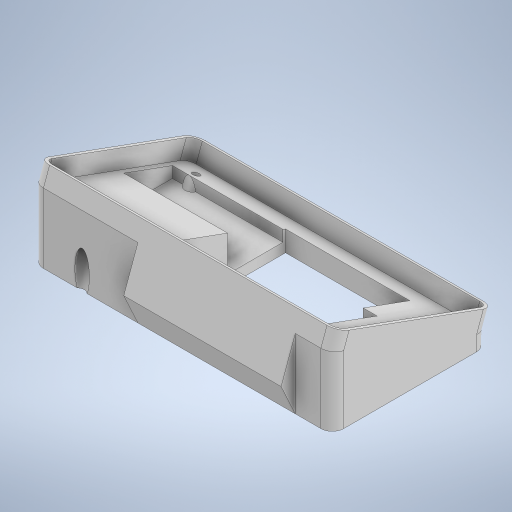
# Autodesk Inventor part: 5inDisplayAdapter-OLED-v3
Saved by Autodesk Inventor 2023 (Build 270158000, 158)
## iProperties
Created: 2024-03-13
Part Number: 5inDisplayAdapter-OLED-v3
Material: Generic
Document SubType Name: Modeling
Designer: incep
Density: 1 g/cm^3
Appearance: Default
Author: incep
## iProperties of the stored document 5inDisplayAdapter_3DPrint.ipt
Created: 2024-03-13
Part Number: 5inDisplayAdapter_3DPrint
Material: Generic
Document SubType Name: Modeling
Designer: incep
Density: 1 g/cm^3
Appearance: Default
Author: incep
Autodesk Inventor part; units mm, degrees
ref_plane "YZ Plane" through (0, 0, 0) normal (1, 0, 0) x (0, 1, 0)
sketch "Sketch1" plane through (0, 0, 0) normal (0, 1, 0) x (-1, 0, 0)
  circle A0 centre (32.29, -13) radius 2.1
  circle A1 centre (-62.1, -13) radius 2.1
  line L0 (72.5, -43) -> (-72.5, -43)
  line L1 (-72.5, -43) -> (-72.5, 32)
  line L2 (-72.5, 32) -> (72.5, 32)
  line L3 (72.5, 32) -> (72.5, -43)
  line L4 (15.095, -33) -> (-44.905, -33)
  line L5 (-44.905, -33) -> (-44.905, 7)
  line L6 (-44.905, 7) -> (15.095, 7)
  line L7 (15.095, 7) -> (15.095, -33)
  line L8 (-62.1, -13) -> (32.29, -13) construction
  point P0 (0, 0)
  point P1 (0, 0)
  point P2 (-14.905, -33)
  point P3 (0, -43)
  point P4 (-44.905, -13)
  point P5 (-72.5, -5.5)
  point P6 (15.095, -13)
  point P7 (-14.905, 7)
  point P8 (0, 32)
  point P9 (-14.905, -13)
  dimension "d1" = 4.2
  dimension "d2" = 60
  dimension "d3" = 40
  dimension "d55" = 25
  dimension "d56" = 10
  dimension "d76" = 145
  dimension "d77" = 75
  dimension "d78" = 94.39
  dimension "d107" = 10.4
  constraints: 18 end point, 8 midpoint, 4 parallel, 3 coincident, 3 horizontal, 2 centre point, 2 perpendicular, 2 vertical alignment, 1 horizontal alignment
  measures "d1" diameter of A0
  measures "d2" distance of L4.start L4.end
  measures "d3" distance between parallel lines of L4 L6
  measures "d55" distance between parallel lines of L2 L6
  measures "d56" distance between parallel lines of L0 L4
  measures "d76" distance of L1.end L2.end
  measures "d77" distance of L0.end L1.end
  measures "d78" distance of L8.start L8.end
  measures "d107" distance from line of L1 A1.centre
extrude "Extrusion1" add sketch "Sketch1" along normal blind 1
sketch "Sketch6" plane through (0, 0, 0) normal (1, 0, 0) x (0, 1, 0)
  line L0 (0, 32) -> (33.618656, 32)
  line L1 (33.618656, 32) -> (6.257045, -43.17541)
  line L2 (0, -43) -> (1, -43)
  line L3 (6.257045, -43.17541) -> (0, -43)
  line L4 (0, -43) -> (0, 32)
  line L5 (0, 32) -> (1, 32)
  line L6 (28.297768, 32) -> (0.9899, -43.027751)
  point P0 (0, 0)
  dimension "d15" = 70
  dimension "d16" = 80
  dimension "d25" = 5
  constraints: 10 end point, 3 point on line, 1 collinear, 1 parallel, 1 perpendicular
  measures "d15" angle of L1 L0
  measures "d16" distance of L0.end L1.end
  measures "d25" distance between parallel lines of L1 L6
extrude "Extrusion2" add sketch "Sketch6" along normal up to surface (72.5 mm away)
sketch "Sketch7" plane through (72.5, 0, 32) normal (1, 0, 0) x (0, 0, -1)
  line L0 (0, 0) -> (75, 0)
  line L1 (75.17541, 6.257045) -> (75, 0)
  line L2 (0, 33.618656) -> (75.17541, 6.257045)
  line L3 (0, 0) -> (0, 33.618656)
  point P0 (32, 0)
extrude "Extrusion3" add sketch "Sketch7" against normal up to surface (145 mm away)
sketch "Sketch8" plane through (-56.5, 6.257045, -43.17541) normal (0, 0.9396926, -0.3420201) x (1, 0, 0)
  line L0 (101.405, -45.009427) -> (41.405, -45.009427) construction
  line L1 (101.405, -7.421722) -> (101.405, -45.009427) construction
  line L2 (41.405, -7.421722) -> (101.405, -7.421722) construction
  line L3 (41.405, -45.009427) -> (41.405, -7.421722) construction
  ellipse E0 centre (24.21, -26.215574) end of major axis (22.11, -26.215574) minor radius 1.973355 construction
  ellipse E1 centre (118.6, -26.215574) end of major axis (116.5, -26.215574) minor radius 1.973355 construction
  line L4 (-3.875, -8.625) -> (118.125, -8.625) construction
  line L5 (118.125, -8.625) -> (118.125, -56.325) construction
  line L6 (118.125, -56.325) -> (-3.875, -56.325) construction
  line L7 (-3.875, -56.325) -> (-3.875, -8.625) construction
  line L8 (-16, 0) -> (129, 0) construction
  circle A0 centre (-3.875, -8.625) radius 1.75
  circle A1 centre (118.125, -8.625) radius 1.75
  circle A2 centre (118.125, -56.325) radius 1.75
  circle A3 centre (-3.875, -56.325) radius 1.75 construction
  line L9 (-16, -80) -> (129, -80)
  line L10 (129, -80) -> (129, 0)
  line L11 (-16, 0) -> (-16, -80)
  line L12 (-3.875, -8.625) -> (8.175, -8.625) construction
  line L13 (8.175, -8.625) -> (8.175, -71.075) construction
  line L14 (8.175, -71.075) -> (-3.875, -71.075) construction
  line L15 (-3.875, -71.075) -> (-3.875, -8.625) construction
  circle A4 centre (8.175, -71.075) radius 1.75
  line L16 (127.5, -1.5) -> (-14.5, -1.5)
  line L17 (-14.5, -1.5) -> (-14.5, -78.5)
  line L18 (-14.5, -78.5) -> (127.5, -78.5)
  line L19 (127.5, -78.5) -> (127.5, -1.5)
  circle A5 centre (8.175, -71.075) radius 3.5
  circle A6 centre (-3.875, -8.625) radius 3.5
  circle A7 centre (118.125, -8.625) radius 3.5
  circle A8 centre (118.125, -56.325) radius 3.5
  line L20 (129, -80) -> (129, 0)
  line L21 (-16, 0) -> (129, 0)
  line L22 (-16, 0) -> (-16, -80)
  line L23 (-16, -80) -> (129, -80)
  line L24 (38.125, -34.727186) -> (108.125, -34.727186)
  line L25 (108.125, -34.727186) -> (108.125, -76)
  line L26 (108.125, -76) -> (38.125, -76)
  line L27 (38.125, -76) -> (38.125, -34.727186)
  line L28 (-12, -12.125) -> (58, -12.125)
  line L29 (58, -12.125) -> (58, -37.125)
  line L30 (58, -37.125) -> (-12, -37.125)
  line L31 (-12, -37.125) -> (-12, -12.125)
  point P0 (56.5, -38.431578)
  point P1 (129, 0)
  point P2 (-16, 0)
  dimension "d22" = 122
  dimension "d23" = 47.7
  dimension "d24" = 3.5
  dimension "d111" = 8.625
  dimension "d112" = 12.125
  dimension "d113" = 10.875
  dimension "d114" = 62.45
  dimension "d115" = 109.95
  dimension "d116" = 8.925
  dimension "d117" = 1.5
  dimension "d118" = 7
  dimension "d119" = 4
  dimension "d120" = 70
  dimension "d121" = 10
  dimension "d122" = 4
  dimension "d123" = 25
  dimension "d124" = 70
  constraints: 40 end point, 9 centre point, 9 coincident, 8 parallel, 7 equal radius, 4 horizontal, 4 perpendicular, 1 tangent, 5 other
  measures "d22" distance of L4.start L4.end
  measures "d23" distance of L4.end L5.end
  measures "d24" diameter of A0
  measures "d111" distance between parallel lines of L8 L4
  measures "d112" distance between parallel lines of L11 L7
  measures "d113" distance between parallel lines of L10 L5
  measures "d114" distance of L12.end L13.end
  measures "d115" distance from line of L5.end L13
  measures "d116" distance between parallel lines of L9 L14
  measures "d117" distance between parallel lines of L10 L19
  measures "d118" diameter of A6
  measures "d119" distance between parallel lines of L26 L23
  measures "d120" distance of L24.start L24.end
  measures "d121" distance from line of L25 L5.end
  measures "d122" distance between parallel lines of L22 L31
  measures "d123" distance of L28.end L29.end
  measures "d124" distance of L29.end L30.end
extrude "Extrusion4" [suppressed]
extrude "Extrusion5" cut sketch "Sketch1" along normal blind 40 contours A0 | A1
ref_plane "Work Plane3" through (0, 5, 0) normal (0, -1, 0) x (1, 0, 0)
sketch "Sketch10" plane through (0, 5, 0) normal (0, -1, 0) x (1, 0, 0)
  circle A0 centre (62.1, -13) radius 2.1 projected
  circle A1 centre (-32.29, -13) radius 2.1 projected
  circle A2 centre (62.1, -13) radius 3.75
  circle A3 centre (-32.29, -13) radius 3.75
  point P0 (0, 0)
  dimension "d35" = 7.5
  constraints: 2 centre point, 2 coincident, 1 equal radius
  measures "d35" diameter of A2
extrude "Extrusion7" cut sketch "Sketch10" against normal blind 40 contours A0 | A1 | A2 | A3
extrude "Extrusion9" cut sketch "Sketch1" along normal blind 40 contours L4 L5 L6 L7
extrude "Extrusion10" [suppressed]
fillet "Fillet1" [suppressed]
sketch "Sketch18" plane through (-32.29, 5, -13) normal (0, 1, 0) x (1, 0, 0)
  line L0 (33.79, -4.710679) -> (-36.21, -4.710679)
  line L1 (-36.21, -4.710679) -> (-36.21, 18.781637)
  line L2 (-36.21, 18.781637) -> (33.79, 18.781637)
  line L3 (33.79, 18.781637) -> (33.79, -4.710679)
  line L4 (13.915, -41.24123) -> (13.915, -2.457471)
  line L5 (13.915, -2.457471) -> (83.915, -2.457471)
  line L6 (83.915, -2.457471) -> (83.915, -41.24123)
  line L7 (83.915, -41.24123) -> (13.915, -41.24123)
  point P0 (32.29, -13)
  point P1 (13.915, -4.710679)
  point P2 (33.79, -2.457471)
extrude "Extrusion17" cut sketch "Sketch18" along normal blind 70
ref_plane "Work Plane6" through (-72.5, 4.37766, -42.491369) normal (0, 0.9396926, -0.3420201) x (1, 0, 0)
sketch "Sketch19" plane through (-72.5, 4.37766, -42.491369) normal (0, 0.9396926, -0.3420201) x (1, 0, 0)
  circle A0 centre (12.125, -8.625) radius 3.5 projected
  circle A1 centre (24.175, -71.075) radius 3.5 projected
  circle A2 centre (134.125, -56.325) radius 3.5 projected
  circle A3 centre (134.125, -8.625) radius 3.5 projected
  point P0 (72.5, -38.431578)
extrude "Extrusion18" cut sketch "Sketch19" against normal blind 70
extrude "Extrusion19" cut sketch "Sketch8" against normal blind 70 contours A0 | A1 | A2 | A4
extrude "Extrusion20" add sketch "Sketch8" against normal up to surface contours A6 surface through (-32.29, 5, -13) normal (0, -1, 0)
extrude "Extrusion21" add sketch "Sketch8" along normal blind 8.65 contours L11 L21 L10 L9
fillet "Fillet6" radius 4 4 edges at (-71, 10.8342, -43.2451) (71, 10.8342, -43.2451) (71, 37.1698, 29.1112) (-71, 37.1698, 29.1112)
fillet "Fillet7" radius 5.5 8 edges at (-72.5, 10.3212, -44.6546) (-72.5, 3.1285, -43.0877) (-72.5, 37.6828, 30.5208) (-72.5, 16.8093, 32) (72.5, 16.8093, 32) (72.5, 37.6828, 30.5208) (72.5, 3.1285, -43.0877) (72.5, 10.3212, -44.6546)
sketch "Sketch20" plane through (-67, 33.105626, 30.590461) normal (0, 0.9396926, -0.3420201) x (1, 0, 0)
  line L0 (45.625, 20.615041) -> (121.625, 20.615041)
  line L1 (121.625, 20.615041) -> (121.625, -1.5)
  line L2 (121.625, -1.5) -> (45.625, -1.5)
  line L3 (45.625, -1.5) -> (45.625, 20.615041)
  line L4 (48.625, 2.5) -> (48.625, 41.375)
  line L5 (118.625, 43.772814) -> (118.625, 2.5)
  line L6 (0, -1.5) -> (134, -1.5)
  line L7 (48.625, 1.5) -> (118.625, 1.5)
  line L8 (118.625, 2.5) -> (48.625, 2.5)
  line L9 (48.625, 2.5) -> (48.625, 1.5)
  line L10 (118.625, 2.5) -> (118.625, 1.5)
  point P0 (67, 40.068422)
  point P1 (118.625, 20.615041)
  point P2 (48.625, 20.615041)
  dimension "d138" = 3
  dimension "d139" = 3
  dimension "d141" = 3
  constraints: 14 end point, 3 perpendicular, 2 horizontal, 2 parallel, 2 vertical, 1 collinear
  measures "d138" distance between parallel lines of L3 L4
  measures "d139" distance between parallel lines of L1 L5
  measures "d141" distance between parallel lines of L7 L2
extrude "Extrusion22" cut sketch "Sketch20" against normal blind 20 contours L0 L5 L8 L4 | L8 L10 L7 L9
extrude "Extrusion23" add sketch "Sketch20" against normal blind 20 contours L0 L4 L9 L7 L10 L5 L1 L2 L3
sketch "Sketch21" plane through (-21.375, 12.335101, 32) normal (-1, 0, 0) x (0, 0, 1)
  line L0 (6.840403, 2.489703) -> (0, -12.335101)
  line L1 (0, 21.283555) -> (0, 0)
  line L2 (0, 0) -> (0, 21.283555)
  line L3 (0, -12.335101) -> (0, 21.283555)
  line L4 (0, -12.335101) -> (0, -12.335101)
  line L5 (0, 21.283555) -> (0, -12.335101)
  line L6 (0, 0) -> (6.840403, 2.489703)
  line L7 (-5.168309, 19.402445) -> (-70.0071, -4.196945)
  point P0 (-32, -12.335101)
  point P1 (0, 0)
  point P2 (0, 0)
  point P3 (0, -12.335101)
  point P4 (0, 0)
  constraints: 4 end point, 1 parallel
extrude "Extrusion24" add sketch "Sketch21" against normal up to surface (76 mm away)
body "Solid1"
